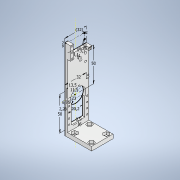
# Autodesk Inventor part: Support AX 12A
Saved by Autodesk Inventor 2022 (Build 260153000, 153)
## iProperties
Created: 2022-01-08
Part Number: Support AX 12A
Material: Générique
Document SubType Name: Modeling
Designer: victo
Density: 1 g/cm^3
Appearance: Par défaut
Source: UnKnown
Author: victo
Autodesk Inventor part; units mm, degrees
ref_plane "YZ Plane" through (0, 0, 0) normal (1, 0, 0) x (0, 1, 0)
ref_plane "XZ Plane" through (0, 0, 0) normal (0, 1, 0) x (-1, 0, 0)
ref_plane "Plan de construction4" through (0, 0, 21) normal (0, 0, 1) x (1, 0, 0)
sketch "Esquisse" plane through (0, 0, 21) normal (0, 0, 1) x (1, 0, 0)
  circle A0 centre (0, 0) radius 11.5
  line L0 (16, -11.5) -> (-16, -11.5) construction
  line L1 (-16, -11.5) -> (-16, 38.5)
  line L2 (-16, 38.5) -> (16, 38.5)
  line L3 (16, 38.5) -> (16, -11.5)
  line L4 (0, 0) -> (-13.5, 6.75) construction
  circle A1 centre (-13.5, 6.75) radius 1.1
  line L5 (-13.5, 6.75) -> (-13.5, 14.75) construction
  line L6 (-13.5, 14.75) -> (-13.5, 22.75) construction
  line L7 (-13.5, 22.75) -> (-13.5, 30.75) construction
  circle A2 centre (-13.5, 30.75) radius 1.1
  circle A3 centre (-13.5, 22.75) radius 1.1
  circle A4 centre (-13.5, 14.75) radius 1.1
  line L8 (-22.4, 0) -> (22.4, 0) construction
  line L9 (10.1, 32.6) -> (10.1, 5.4991)
  line L10 (-10.1, 5.4991) -> (-10.1, 32.6)
  line L11 (-10.1, 32.6) -> (10.1, 32.6)
  line L12 (16, -11.5) -> (0, 0) construction
  line L13 (-16, -11.5) -> (0, 0) construction
  line L14 (10.1, 5.4991) -> (-10.1, 5.4991) construction
  line L15 (16, 38.5) -> (-16, 38.5)
  line L16 (-16, 38.5) -> (-16, 39.5)
  line L17 (-16, 39.5) -> (16, 39.5)
  line L18 (16, 39.5) -> (16, 38.5)
  line L19 (0, -98.8) -> (0, 69.55) construction
  circle A5 centre (13.5, 6.75) radius 1.1
  circle A6 centre (13.5, 30.75) radius 1.1
  circle A7 centre (13.5, 22.75) radius 1.1
  circle A8 centre (13.5, 14.75) radius 1.1
  line L20 (-16, -11.5) -> (16, -11.5) construction
  line L21 (16, -11.5) -> (16, -16.5)
  line L22 (16, -16.5) -> (-16, -16.5)
  line L23 (-16, -16.5) -> (-16, -11.5)
  line L24 (16, 39.5) -> (-16, 39.5)
  line L25 (-16, 39.5) -> (-16, 45.5)
  line L26 (-16, 45.5) -> (16, 45.5)
  line L27 (16, 45.5) -> (16, 39.5)
  line L28 (16, -16.5) -> (-16, -16.5)
  line L29 (-16, -16.5) -> (-16, -59)
  line L30 (-16, -59) -> (-11.5, -59)
  line L31 (16, -59) -> (16, -16.5)
  circle A9 centre (0, -50) radius 1.55
  line L32 (13.5, -56.75) -> (-13.5, -56.75) construction
  line L33 (-13.5, -56.75) -> (-13.5, -64.75) construction
  line L34 (-13.5, -64.75) -> (-13.5, -72.75) construction
  line L35 (-13.5, -72.75) -> (13.5, -72.75) construction
  line L36 (13.5, -72.75) -> (13.5, -64.75) construction
  line L37 (13.5, -64.75) -> (13.5, -56.75) construction
  circle A10 centre (13.5, -72.75) radius 1.1
  circle A11 centre (13.5, -64.75) radius 1.1
  circle A12 centre (13.5, -56.75) radius 1.1
  circle A13 centre (-13.5, -56.75) radius 1.1
  circle A14 centre (-13.5, -64.75) radius 1.1
  circle A15 centre (-13.5, -72.75) radius 1.1
  line L38 (16, -54.75) -> (11.5, -54.75)
  line L39 (11.5, -54.75) -> (11.5, -59)
  line L40 (-11.5, -59) -> (-11.5, -54.75)
  line L41 (-11.5, -54.75) -> (-16, -54.75)
  line L42 (-11.5, -59) -> (16, -59)
  line L43 (-11.5, -59) -> (-11.5, -74.75)
  line L44 (-11.5, -74.75) -> (-16, -74.75)
  line L45 (-16, -74.75) -> (-16, -59)
  line L46 (0, -50) -> (11, -50) construction
  line L47 (11, -50) -> (11, -39) construction
  circle A16 centre (11, -50) radius 1.55
  circle A17 centre (11, -39) radius 1.55
  point P0 (0, -11.5)
  point P1 (16, -11.5)
  dimension "d107" = 23
  dimension "d133" = 6.75
  dimension "d135" = 2.2
  dimension "d137" = 8
  dimension "d138" = 20.2
  dimension "d160" = 50
  dimension "d161" = 5.9
  dimension "d162" = 32
  dimension "d163" = 11.5
  dimension "d169" = 5
  dimension "d224" = 1
  dimension "d225" = 6
  dimension "d240" = 13.5
  dimension "d242" = 32
  dimension "d243" = 3.1
  dimension "d249" = 50
  dimension "d250" = 6.75
  dimension "d251" = 8
  dimension "d252" = 2.2
  dimension "d253" = 2
  dimension "d254" = 2
  dimension "d255" = 9
  dimension "d258" = 2
  dimension "d261" = 3.1
  dimension "d263" = 11
  dimension "d264" = 11
  constraints: 92 end point, 18 centre point, 13 coincident, 13 perpendicular, 12 parallel, 10 point on line, 9 equal radius, 9 horizontal, 7 equal length, 5 collinear, 5 vertical, 4 symmetric about line, 2 point on circle, 4 other
  measures "d107" diameter of A0
  measures "d133" vertical distance of L4.start L4.end
  measures "d135" diameter of A1
  measures "d137" distance of L5.start L5.end
  measures "d138" distance between parallel lines of L10 L9
  measures "d160" distance between parallel lines of L2 L0
  measures "d161" distance between parallel lines of L2 L11
  measures "d162" distance between parallel lines of L3 L1
  measures "d163" distance from line of L0 point (0, 0)
  measures "d169" distance between parallel lines of L22 L0
  measures "d224" distance between parallel lines of L17 L2
  measures "d225" distance between parallel lines of L26 L17
  measures "d240" distance from line of L19 L5.end
  measures "d242" distance of L29.end L31.start
  measures "d243" diameter of A9
  measures "d249" distance of L4.start L46.start
  measures "d250" distance from line of L46.start L32
  measures "d251" distance of L36.end L32.start
  measures "d252" diameter of A10
  measures "d253" distance from line of L38 L32.start
  measures "d254" distance from line of L39 L32.start
  measures "d255" distance from line of L30 L46.start
  measures "d258" distance from line of L44 L34.end
  measures "d261" diameter of A16
  measures "d263" distance from line of L47.end L46
  measures "d264" distance of L46.start L46.end
extrude "Face fixation moteur" add sketch "Esquisse" against normal blind 4 contours L1 L2 L3 L21 L22 L23 | L16 L17 L18 L2 | L22 L31 L38 L39 L42 L40 L41 L29 | L41 L40 L30 L29 | L31 L42 L39 L38
extrude "Creux moteur" [suppressed]
extrude "Rai basl" add sketch "Esquisse" against normal blind 40 contours L25 L26 L27 L17
sketch "Esquisse16" plane through (-16, 39.5, 17) normal (0, -1, 0) x (1, 0, 0)
  line L0 (0, 0) -> (0, -36) projected
  line L1 (32, -36) -> (0, -36) projected
  line L2 (32, 0) -> (32, -36) projected
  line L3 (5, -6) -> (27, -6) construction
  line L4 (27, -6) -> (27, -31) construction
  line L5 (27, -31) -> (5, -31) construction
  line L6 (5, -31) -> (5, -6) construction
  line L7 (0, 0) -> (0, -36) projected
  line L8 (0, -1) -> (5, -6) construction
  line L9 (5, -31) -> (0, -36) construction
  line L10 (0, -36) -> (32, -36) projected
  line L11 (27, -31) -> (32, -36) construction
  circle A0 centre (5, -6) radius 2.1
  circle A1 centre (27, -6) radius 2.1
  circle A2 centre (27, -31) radius 2.1
  circle A3 centre (5, -31) radius 2.1
  line L12 (6.1207, -10.1826) -> (1.9381, -9.0619)
  line L13 (1.9381, -9.0619) -> (0.8174, -4.8793)
  line L14 (0.8174, -4.8793) -> (3.8793, -1.8174)
  line L15 (3.8793, -1.8174) -> (8.0619, -2.9381)
  line L16 (8.0619, -2.9381) -> (9.1826, -7.1207)
  line L17 (9.1826, -7.1207) -> (6.1207, -10.1826)
  line L18 (9.1826, -29.8793) -> (8.0619, -34.0619)
  line L19 (8.0619, -34.0619) -> (3.8793, -35.1826)
  line L20 (3.8793, -35.1826) -> (0.8174, -32.1207)
  line L21 (0.8174, -32.1207) -> (1.9381, -27.9381)
  line L22 (1.9381, -27.9381) -> (6.1207, -26.8174)
  line L23 (6.1207, -26.8174) -> (9.1826, -29.8793)
  line L24 (25.8793, -26.8174) -> (30.0619, -27.9381)
  line L25 (30.0619, -27.9381) -> (31.1826, -32.1207)
  line L26 (31.1826, -32.1207) -> (28.1207, -35.1826)
  line L27 (28.1207, -35.1826) -> (23.9381, -34.0619)
  line L28 (23.9381, -34.0619) -> (22.8174, -29.8793)
  line L29 (22.8174, -29.8793) -> (25.8793, -26.8174)
  line L30 (22.8174, -7.1207) -> (23.9381, -2.9381)
  line L31 (23.9381, -2.9381) -> (28.1207, -1.8174)
  line L32 (28.1207, -1.8174) -> (31.1826, -4.8793)
  line L33 (31.1826, -4.8793) -> (30.0619, -9.0619)
  line L34 (30.0619, -9.0619) -> (25.8793, -10.1826)
  line L35 (25.8793, -10.1826) -> (22.8174, -7.1207)
  line L36 (7.6517, -8.6517) -> (24.3483, -8.6517) construction
  line L37 (24.3483, -8.6517) -> (24.3483, -28.3483) construction
  line L38 (24.3483, -28.3483) -> (7.6517, -28.3483) construction
  line L39 (7.6517, -28.3483) -> (7.6517, -8.6517) construction
  line L40 (32, 4) -> (0, 4) projected
  line L41 (26.1, 4) -> (5.9, 4) projected
  line L42 (5.9, 4) -> (26.1, 4) projected
  line L43 (28.4, 4) -> (30.6, 4) projected
  line L44 (28.4, 4) -> (30.6, 4) projected
  line L45 (1.4, 4) -> (3.6, 4) projected
  line L46 (1.4, 4) -> (3.6, 4) projected
  line L47 (1.4, 4) -> (3.6, 4) projected
  line L48 (1.4, 4) -> (3.6, 4) projected
  line L49 (28.4, 4) -> (30.6, 4) projected
  line L50 (28.4, 4) -> (30.6, 4) projected
  line L51 (32, 0) -> (32, -36) projected
  line L52 (0, 0) -> (0, -36) projected
  line L53 (32, -1) -> (27, -6) construction
  line L54 (0, -1) -> (32, -1)
  line L55 (0, 0) -> (32, 0) projected
  line L56 (0, 4) -> (32, 4) projected
  point P0 (16, -17)
  dimension "d228" = 5
  dimension "d229" = 5
  dimension "d230" = 4.2
  dimension "d231" = 7.5
  dimension "d232" = 25
  dimension "d233" = 22
  dimension "d245" = 40
  dimension "d246" = 32
  dimension "d248" = 1
  constraints: 74 end point, 8 coincident, 5 point on line, 4 centre point, 4 equal length, 4 midpoint, 4 parallel, 3 equal radius, 3 perpendicular, 2 horizontal, 52 other
  measures "d228" distance between parallel lines of L0 L6
  measures "d229" distance between parallel lines of L1 L5
  measures "d230" diameter of A0
  measures "d231" distance between parallel lines of L17 L14
  measures "d232" distance between parallel lines of L5 L3
  measures "d233" distance between parallel lines of L6 L4
  measures "d245" distance from line of L10 L56.start
  measures "d246" distance of L0.end L1.start
  measures "d248" distance between parallel lines of L54 L55
extrude "Extrusion23" cut sketch "Esquisse16" against normal through all contours A0 | A1 | A2 | A3
extrude "Extrusion24" cut sketch "Esquisse16" against normal blind 4 contours A3 | L12 L13 L14 L15 L16 L17 | L18 L19 L20 L21 L22 L23 | L24 L25 L26 L27 L28 L29 | L30 L31 L32 L33 L34 L35
extrude "Extrusion25" add sketch "Esquisse" against normal blind 8.5 contours L41 L40 L30 L29 | L31 L42 L39 L38 | L30 L43 L44 L45
